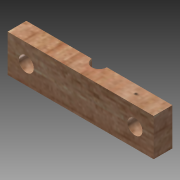
# Autodesk Inventor part: Z_MotorMount_RodHolder_Part2_V2
Saved by Autodesk Inventor 2014 (Build 180170000, 170)
## iProperties
Created: 2013-12-13
Part Number: Z_MotorMount_RodHolder_Part2_V2
Material: Birch
Document SubType Name: Modeling
Designer: Bram
Density: 0.512 g/cm^3
Appearance: Birch - Natural Medium Gloss
Author: Bram
Autodesk Inventor part; units mm, degrees
ref_plane "YZ Plane" through (0, 0, 0) normal (1, 0, 0) x (0, 1, 0)
ref_plane "XZ Plane" through (0, 0, 0) normal (0, 1, 0) x (-1, 0, 0)
ref_plane "XY Plane" through (0, 0, 0) normal (0, 0, 1) x (1, 0, 0)
sketch "Sketch1" plane through (0, 0, 0) normal (0, 1, 0) x (-1, 0, 0)
  line L0 (0, 0) -> (78, 0)
  line L1 (78, 0) -> (78, 20)
  line L2 (78, 20) -> (0, 20)
  line L3 (0, 20) -> (0, 0)
  line L4 (39, 10) -> (68, 10)
  line L5 (39, 10) -> (10, 10)
  circle A0 centre (10, 10) radius 4
  circle A1 centre (68, 10) radius 4
  dimension "d0" = 78
  dimension "d1" = 20
  dimension "d2" = 29
  dimension "d3" = 29
  dimension "d4" = 8
  dimension "d5" = 8
  constraints: 12 end point, 3 equal length, 2 centre point, 2 coincident, 2 perpendicular, 1 horizontal
  measures "d0" distance of L2.end L1.end
  measures "d1" distance of L1.end L0.end
  measures "d2" distance of L4.start L4.end
  measures "d3" distance of L4.start L5.end
  measures "d4" diameter of A0
  measures "d5" diameter of A1
extrude "Extrusion1" add sketch "Sketch1" along normal blind 10
sketch "Sketch2" plane through (-78, 0, 20) normal (0, 0, 1) x (1, 0, 0)
  line L0 (0, 10) -> (78, 10) projected
  circle A0 centre (39, 10) radius 4
  dimension "d8" = 8
  constraints: 1 centre point, 1 midpoint
  measures "d8" diameter of A0
extrude "Extrusion2" cut sketch "Sketch2" against normal blind 20
body "Solid1"
